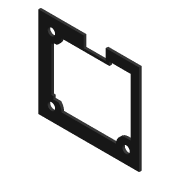
# Autodesk Inventor part: resin_top
Saved by Autodesk Inventor 2015 SP1 (Build 190203100, 203)
## iProperties
Created: 2015-12-07
Part Number: resin_top
Material: Типовые
Document SubType Name: Modeling
Designer: User
Density: 1 g/cm^3
Appearance: По умолчанию
Mass: 0.611168 g
Surface Area: 15.2419 cm^2
Volume: 0.611168 cm^3
Author: User
Autodesk Inventor part; units mm, degrees
ref_plane "YZ Plane" through (0, 0, 0) normal (1, 0, 0) x (0, 1, 0)
ref_plane "XZ Plane" through (0, 0, 0) normal (0, 1, 0) x (-1, 0, 0)
ref_plane "XY Plane" through (0, 0, 0) normal (0, 0, 1) x (1, 0, 0)
sketch "Эскиз1" plane through (0, 0, 0) normal (0, 1, 0) x (-1, 0, 0)
  line L0 (18, -16) -> (-18, -16)
  line L1 (-18, -16) -> (-18, 16)
  line L2 (-18, 16) -> (18, 16)
  line L3 (18, 16) -> (18, -16)
  line L4 (14.82, -12.82) -> (-14.82, -12.82)
  line L5 (-14.82, -12.82) -> (-14.82, 12.82)
  line L6 (-14.82, 12.82) -> (14.82, 12.82)
  line L7 (14.82, 12.82) -> (14.82, -12.82)
  circle A0 centre (14.82, -12.82) radius 1.5
  circle A1 centre (14.82, 12.82) radius 1.5
  circle A2 centre (-14.82, 12.82) radius 1.5
  circle A3 centre (-14.82, -12.82) radius 1.5
  arc A4 (11.9634, -10.02) -> (14.12, -8.8817) centre (14.82, -12.82) ccw
  circle A5 centre (-14.82, -12.82) radius 4
  arc A6 (14.12, 8.8817) -> (12.7129, 9.42) centre (14.82, 12.82) ccw
  arc A7 (-11.0303, 14.1) -> (-16.6, 9.2379) centre (-14.82, 12.82) ccw
  line L8 (14.12, -10.02) -> (1.12, -10.02)
  line L9 (1.12, -10.02) -> (1.12, 9.42)
  line L10 (1.12, 9.42) -> (14.12, 9.42)
  line L11 (14.12, 9.42) -> (14.12, -10.02)
  line L12 (-9.6, 7.9) -> (-16.6, 7.9)
  line L13 (-16.6, 7.9) -> (-16.6, 14.1)
  line L14 (-16.6, 14.1) -> (-9.6, 14.1)
  line L15 (-9.6, 14.1) -> (-9.6, 7.9)
  line L16 (-11.0303, 14.1) -> (-16.6, 14.1)
  line L17 (14.12, 8.8817) -> (14.12, 9.42)
  line L18 (14.12, -8.8817) -> (14.12, -10.02)
  line L19 (11.9634, -10.02) -> (14.12, -10.02)
  circle A8 centre (-13.034, 10.913) radius 1.5
  circle A9 centre (-13.034, 10.913) radius 1.25
  line L20 (20, -18) -> (-20, -18)
  line L21 (-20, -18) -> (-20, 18)
  line L22 (-20, 18) -> (20, 18)
  line L23 (20, 18) -> (20, -18)
  line L24 (-10.82, -12.82) -> (-10.82, -16)
  line L25 (-14.82, -8.82) -> (-18, -8.82)
  line L26 (10.82, -12.82) -> (10.82, -16)
  line L27 (14.82, -8.82) -> (18, -8.82)
  line L28 (14.82, 8.82) -> (18, 8.82)
  line L29 (10.82, 12.82) -> (10.82, 16)
  line L30 (-18, 8.82) -> (-16.6, 8.82)
  line L31 (-10.82, 16) -> (-10.82, 14.1)
  line L32 (-10.82, 14.1) -> (-11.0303, 14.1)
  line L33 (-16.6, 9.2379) -> (-16.6, 8.82)
  line L34 (3.5, 16) -> (3.5, 12.6)
  line L35 (3.5, 12.6) -> (-8.2, 12.6)
  line L36 (-8.2, 12.6) -> (-8.2, 16)
  line L37 (-6.7, 18) -> (-6.7, 13.6)
  line L38 (-6.7, 13.6) -> (2, 13.6)
  line L39 (2, 13.6) -> (2, 18)
  line L40 (3.5, 16) -> (3.5, 12.6)
  line L41 (-8.2, 12.6) -> (3.5, 12.6)
  line L42 (-8.2, 12.6) -> (-8.2, 16)
  line L43 (-8.2, 16) -> (-6.7, 16)
  line L44 (-6.7, 16) -> (-6.7, 13.6)
  line L45 (-6.7, 13.6) -> (2, 13.6)
  line L46 (2, 13.6) -> (2, 16)
  line L47 (2, 16) -> (3.5, 16)
  line L48 (-10.82, 14.1) -> (-8.2, 14.1)
  line L49 (-8.2, 14.1) -> (-8.2, 16)
  line L50 (3.5, 12.6) -> (10.8261, 12.6)
  line L51 (10.8261, 12.6) -> (10.82, 12.82)
  line L52 (10.82, 12.82) -> (3.5, 12.82)
  line L53 (3.5, 12.82) -> (3.5, 12.6)
  line L54 (-16.6, 7.9) -> (-16.6, -8.82)
  line L55 (-16.6, -8.82) -> (-18, -8.82)
  line L56 (-18, -8.82) -> (-18, 8.82)
  point P0 (0, 0)
  dimension "d0" = 36
  dimension "d1" = 32
  dimension "d2" = 3.18
  dimension "d3" = 3.18
  dimension "d4" = 3.18
  dimension "d5" = 3.18
  dimension "d6" = 3
  dimension "d7" = 3
  dimension "d8" = 3
  dimension "d9" = 3
  dimension "d10" = 8
  dimension "d11" = 8
  dimension "d12" = 8
  dimension "d13" = 8
  dimension "d14" = 2.8
  dimension "d15" = 0.7
  dimension "d16" = 3.4
  dimension "d17" = 13
  dimension "d18" = 1.9
  dimension "d19" = 1.4
  dimension "d20" = 7
  dimension "d21" = 6.2
  dimension "d22" = 4.966
  dimension "d23" = 5.087
  dimension "d24" = 3
  dimension "d25" = 2.5
  dimension "d26" = 2
  dimension "d27" = 2
  dimension "d28" = 2
  dimension "d29" = 2
  dimension "d30" = 4
  dimension "d31" = 4
  dimension "d32" = 16
  dimension "d33" = 11.3
  dimension "d34" = 1
  dimension "d35" = 1.5
  dimension "d36" = 1.5
  dimension "d37" = 2.4
  constraints: 114 end point, 36 point on line, 22 perpendicular, 13 point on circle, 11 parallel, 10 centre point, 10 coincident, 9 collinear, 5 horizontal, 3 tangent, 2 vertical
  measures "d0" distance of L0.start L0.end
  measures "d1" distance of L0.end L1.end
  measures "d2" distance between parallel lines of L3 L7
  measures "d3" distance between parallel lines of L2 L6
  measures "d4" distance between parallel lines of L1 L5
  measures "d5" distance between parallel lines of L0 L4
  measures "d6" diameter of A0
  measures "d7" diameter of A1
  measures "d8" diameter of A2
  measures "d9" diameter of A3
  measures "d10" diameter of A4
  measures "d11" diameter of A5
  measures "d12" diameter of A6
  measures "d13" diameter of A7
  measures "d14" distance between parallel lines of L4 L8
  measures "d15" distance between parallel lines of L7 L11
  measures "d16" distance between parallel lines of L6 L10
  measures "d17" distance of L9.end L10.end
  measures "d18" distance between parallel lines of L2 L14
  measures "d19" distance between parallel lines of L1 L13
  measures "d20" distance of L12.start L12.end
  measures "d21" distance of L14.end L12.start
  measures "d22" distance from line of L1 point (-13.034, 10.913)
  measures "d23" distance from line of L2 point (-13.034, 10.913)
  measures "d24" diameter of A8
  measures "d25" diameter of A9
  measures "d26" distance between parallel lines of L20 L0
  measures "d27" distance between parallel lines of L23 L3
  measures "d28" distance between parallel lines of L2 L22
  measures "d29" distance between parallel lines of L21 L1
  measures "d30" distance between parallel lines of L30 L6
  measures "d31" distance between parallel lines of L31 L5
  measures "d32" distance between parallel lines of L3 L39
  measures "d33" distance between parallel lines of L1 L37
  measures "d34" distance between parallel lines of L35 L38
  measures "d35" distance between parallel lines of L34 L39
  measures "d36" distance between parallel lines of L36 L37
  measures "d37" distance between parallel lines of L38 L2
extrude "Выдавливание1" add sketch "Эскиз1" along normal blind 1 contours L0 A4 L3 A6 L2 L39 L22 L23 L20 L21 L37 A7 L1 A5 | L26 A4 L0 | L0 L24 L4 L26 | L0 A5 L24 | A4 L4 A0 L7 L3 L0 | L0 A4 | A4 L8 L11 L7 A0 L4 | A5 L0 | L0 A5 L1 L5 A3 L4 | L4 A3 L5 A5 | A4 L3 L0 | A0 L7 L4 | L4 L7 A0 | L0 L1 A5 | A3 L5 L4 | L4 L5 A3 | A5 L1 L25 | L3 A4 | A5 L1 | A4 L27 L3 | L7 L28 L3 L27 | A6 L11 L10 L6 A1 L7 | L7 A1 L6 A6 L2 L3 | A6 L3 L28 | L14 L13 A7 L1 L2 A2 | A2 L14 | L30 L1 A7 L13 | A1 L6 L7 | L7 L6 A1 | L3 A6 | L36 L2 L37 L38 L39 L34 L6 | A7 L1 | A6 L2 L3 | L29 L2 A6 | A7 L2 L31 L14 | L1 L2 A7 | L2 A6 | L2 A7
extrude "Выдавливание2" add sketch "Эскиз1" along normal blind 1 contours L25 L1 L30 L13 L54 | L14 L13 A7 L1 L2 A2 | A2 L14 | L30 L1 A7 L13 | L50 L34 L6 A6 | L36 L2 L37 L38 L39 L34 L6 | L6 L34 L35 L36 | L14 L31 L2 L36 L48 | L6 L34 L2 L29 | A7 L2 L31 L14 | L1 L2 A7
extrude "Выдавливание3" cut sketch "Эскиз1" along normal blind 1 contours A0 L7 L4 | L4 L7 A0 | A3 L5 L4 | L4 L5 A3 | A1 L6 L7 | L7 L6 A1
equation "\"d6\" = d9"
equation "\"d7\" = d9"
equation "\"d8\" = d9"
